Forms (Autodesk Fusion 360 design; units mm, degrees)
Autodesk Fusion 360 part; units mm, degrees
note: some values were not read from the file. Set by a fixed rule: which sketch regions a step uses.
sketch "Sketch1" plane through (0, 0, 0) normal (0, 0, 1) x (1, 0, 0)
  circle A0 centre (0, 0) radius 40
  circle A1 centre (150, 0) radius 40
  circle A2 centre (150, 0) radius 22.5
  line L0 (220, 40) -> (290, 40)
  line L1 (290, 40) -> (290, -30)
  line L2 (290, -30) -> (220, -30)
  line L3 (220, -30) -> (220, 40)
  line L4 (393.5132, 46.2887) -> (356.9124, 18.1157)
  line L5 (356.9124, 18.1157) -> (363.0105, -27.668)
  line L6 (363.0105, -27.668) -> (405.7094, -45.2787)
  line L7 (405.7094, -45.2787) -> (442.3102, -17.1057)
  line L8 (442.3102, -17.1057) -> (436.2121, 28.678)
  line L9 (436.2121, 28.678) -> (393.5132, 46.2887)
  point P0 (399.6113, 0.505)
  dimension "d1" = 80
  dimension "d2" = 80
  dimension "d3" = 45
  dimension "d4" = 70
  dimension "d5" = 70
  dimension "d6" = 40
  constraint coincident A0.centre origin
  constraint concentric A1 A2
  constraint horizontal L0
  constraint vertical L1
  constraint horizontal L2
  constraint vertical L3
  measures "d1" diameter of A0
  measures "d2" diameter of A1
  measures "d3" diameter of A2
  measures "d4" distance of L0.start L0.end
  measures "d5" distance of L0.start L2.end
  measures "d6" distance of P0 L9
extrude "Extrude1" add sketch "Sketch1" along normal blind 0.6 makes body 1 at (183.934, -3.105, 0) makes body 2 at (243.3333, 16.6667, 0) makes body 3 at (9.4847, -14.2223, 0) makes body 4 at (387.411, -8.886, 0)
sketch "Sketch2" plane through (0, 0, 0) normal (0, 0, 1) x (1, 0, 0)
  line L0 (-102.8513, 50) -> (-56.4512, -30.3672)
  line L1 (-56.4512, -30.3672) -> (-149.2513, -30.3672)
  line L2 (-149.2513, -30.3672) -> (-102.8513, 50)
  spline S0 degree 3 poles (-260.7978, 3.4174) (-243.8859, 0.3631) (-229.7421, -4.5389) (-219.4989, -12.0435) knots 0 0 0 0 1 1 1 1
  line L3 (-219.4989, -12.0435) -> (-224.2157, -12.0435)
  spline S1 degree 3 poles (-224.2157, -12.0435) (-234.8465, -6.8357) (-247.7436, -3.4645) (-262.3437, -1.4752) knots 0 0 0 0 1 1 1 1
  spline S2 degree 3 poles (-262.3437, -1.4752) (-262.9281, -1.3955) (-263.5204, -1.5157) (-264.038, -1.7987) knots 0 0 0 0 1 1 1 1
  spline S3 degree 3 poles (-264.038, -1.7987) (-267.9394, -3.9316) (-272.0672, -4.6023) (-276.5199, -4.8113) knots 0 0 0 0 1 1 1 1
  spline S4 degree 3 poles (-276.5199, -4.8113) (-279.9376, -4.9718) (-283.9097, -8.2703) (-284.0145, -9.2137) knots 0 0 0 0 1 1 1 1
  spline S5 degree 3 poles (-284.0145, -9.2137) (-286.3248, -30.0083) (-292.115, -40.2015) (-306.2361, -45.3236) knots 0 0 0 0 1 1 1 1
  spline S6 degree 3 poles (-306.2361, -45.3236) (-317.133, -48.2569) (-327.3208, -52.6393) (-337.0006, -58.0591) knots 0 0 0 0 1 1 1 1
  spline S7 degree 3 poles (-337.0006, -58.0591) (-336.8531, -67.2004) (-337.3497, -73.1816) (-338.2267, -77.2973) knots 0 0 0 0 1 1 1 1
  spline S8 degree 3 poles (-338.2267, -77.2973) (-338.2811, -77.5527) (-338.6377, -77.5743) (-338.7228, -77.3273) knots 0 0 0 0 1 1 1 1
  spline S9 degree 3 poles (-338.7228, -77.3273) (-340.0463, -73.4885) (-340.059, -67.9976) (-339.4115, -61.6754) knots 0 0 0 0 1 1 1 1
  spline S10 degree 3 poles (-339.4115, -61.6754) (-340.196, -70.3905) (-341.2782, -77.6979) (-342.7181, -83.3138) knots 0 0 0 0 1 1 1 1
  spline S11 degree 3 poles (-342.7181, -83.3138) (-342.7818, -83.562) (-343.1125, -83.6149) (-343.2471, -83.3969) knots 0 0 0 0 1 1 1 1
  spline S12 degree 3 poles (-343.2471, -83.3969) (-344.9354, -80.664) (-344.3802, -73.7091) (-341.8224, -62.9855) knots 0 0 0 0 1 1 1 1
  spline S13 degree 3 poles (-341.8224, -62.9855) (-343.6654, -68.0442) (-345.273, -72.8197) (-345.9627, -77.1363) knots 0 0 0 0 1 1 1 1
  spline S14 degree 3 poles (-345.9627, -77.1363) (-346.6868, -81.6681) (-347.3474, -85.3887) (-348.5401, -86.6625) knots 0 0 0 0 1 1 1 1
  spline S15 degree 3 poles (-348.5401, -86.6625) (-348.7985, -86.9386) (-349.2453, -86.9301) (-349.4925, -86.644) knots 0 0 0 0 1 1 1 1
  spline S16 degree 3 poles (-349.4925, -86.644) (-350.6585, -85.2949) (-350.8832, -82.2734) (-349.7887, -78.0269) knots 0 0 0 0 1 1 1 1
  spline S17 degree 3 poles (-349.7887, -78.0269) (-348.5261, -73.1287) (-346.4266, -68.1391) (-344.3905, -62.8804) knots 0 0 0 0 1 1 1 1
  spline S18 degree 3 poles (-344.3905, -62.8804) (-346.9247, -68.2647) (-349.2979, -72.9995) (-351.402, -76.6499) knots 0 0 0 0 1 1 1 1
  spline S19 degree 3 poles (-351.402, -76.6499) (-351.4977, -76.816) (-351.7419, -76.8027) (-351.8199, -76.6275) knots 0 0 0 0 1 1 1 1
  spline S20 degree 3 poles (-351.8199, -76.6275) (-352.271, -75.6135) (-352.5103, -74.3407) (-351.9899, -72.9432) knots 0 0 0 0 1 1 1 1
  spline S21 degree 3 poles (-351.9899, -72.9432) (-350.8238, -69.8118) (-348.3529, -65.5636) (-346.6966, -62.8804) knots 0 0 0 0 1 1 1 1
  spline S22 degree 3 poles (-346.6966, -62.8804) (-348.4004, -64.8165) (-350.018, -66.7369) (-351.5361, -68.6392) knots 0 0 0 0 1 1 1 1
  spline S23 degree 3 poles (-351.5361, -68.6392) (-351.6431, -68.7732) (-351.8603, -68.697) (-351.8581, -68.5254) knots 0 0 0 0 1 1 1 1
  spline S24 degree 3 poles (-351.8581, -68.5254) (-351.8238, -65.7106) (-348.2696, -62.1588) (-345.7532, -57.9018) knots 0 0 0 0 1 1 1 1
  spline S25 degree 3 poles (-345.7532, -57.9018) (-343.353, -53.8412) (-343.0694, -48.7587) (-343.0278, -43.5938) knots 0 0 0 0 1 1 1 1
  spline S26 degree 3 poles (-343.0278, -43.5938) (-342.8346, -36.7125) (-341.0335, -30.7038) (-337.6296, -25.5647) knots 0 0 0 0 1 1 1 1
  spline S27 degree 3 poles (-337.6296, -25.5647) (-339.0225, -27.1571) (-340.4289, -28.1941) (-341.8523, -28.5418) knots 0 0 0 0 1 1 1 1
  spline S28 degree 3 poles (-341.8523, -28.5418) (-342.2112, -28.6295) (-342.5542, -28.3294) (-342.4991, -27.9641) knots 0 0 0 0 1 1 1 1
  spline S29 degree 3 poles (-342.4991, -27.9641) (-341.9561, -24.3647) (-337.6367, -20.0679) (-333.2801, -15.7644) knots 0 0 0 0 1 1 1 1
  spline S30 degree 3 poles (-333.2801, -15.7644) (-338.7374, -21.2252) (-344.2145, -25.6888) (-349.7179, -28.8857) knots 0 0 0 0 1 1 1 1
  spline S31 degree 3 poles (-349.7179, -28.8857) (-349.9461, -29.0183) (-350.2082, -28.778) (-350.0965, -28.5389) knots 0 0 0 0 1 1 1 1
  spline S32 degree 3 poles (-350.0965, -28.5389) (-347.7567, -23.5322) (-342.0571, -19.1377) (-336.2153, -14.7685) knots 0 0 0 0 1 1 1 1
  spline S33 degree 3 poles (-336.2153, -14.7685) (-339.0427, -17.3429) (-342.3108, -19.242) (-345.5638, -21.431) knots 0 0 0 0 1 1 1 1
  spline S34 degree 3 poles (-345.5638, -21.431) (-349.1875, -23.8693) (-351.6975, -26.9643) (-356.2946, -27.6713) knots 0 0 0 0 1 1 1 1
  spline S35 degree 3 poles (-356.2946, -27.6713) (-356.6004, -27.7184) (-356.8157, -27.374) (-356.6379, -27.1208) knots 0 0 0 0 1 1 1 1
  spline S36 degree 3 poles (-356.6379, -27.1208) (-353.9362, -22.2172) (-346.509, -17.533) (-339.4126, -13.5629) knots 0 0 0 0 1 1 1 1
  spline S37 degree 3 poles (-339.4126, -13.5629) (-348.5941, -18.5484) (-357.9988, -24.0418) (-362.7798, -25.3474) knots 0 0 0 0 1 1 1 1
  spline S38 degree 3 poles (-362.7798, -25.3474) (-363.1677, -25.4533) (-363.538, -25.1083) (-363.4388, -24.7186) knots 0 0 0 0 1 1 1 1
  spline S39 degree 3 poles (-363.4388, -24.7186) (-362.6459, -21.6042) (-354.2725, -17.3356) (-344.3382, -12.8296) knots 0 0 0 0 1 1 1 1
  spline S40 degree 3 poles (-344.3382, -12.8296) (-353.2052, -16.5242) (-363.2289, -20.8213) (-366.6642, -21.6868) knots 0 0 0 0 1 1 1 1
  spline S41 degree 3 poles (-366.6642, -21.6868) (-368.0791, -22.1148) (-369.2325, -22.1652) (-370.2679, -22.045) knots 0 0 0 0 1 1 1 1
  spline S42 degree 3 poles (-370.2679, -22.045) (-370.7274, -21.9917) (-370.9442, -21.4371) (-370.6353, -21.0928) knots 0 0 0 0 1 1 1 1
  spline S43 degree 3 poles (-370.6353, -21.0928) (-367.6264, -17.7386) (-355.2227, -14.2376) (-345.9626, -10.7862) knots 0 0 0 0 1 1 1 1
  spline S44 degree 3 poles (-345.9626, -10.7862) (-355.4959, -13.5245) (-364.6122, -16.3755) (-370.4639, -17.8942) knots 0 0 0 0 1 1 1 1
  spline S45 degree 3 poles (-370.4639, -17.8942) (-371.8406, -18.1302) (-373.6743, -18.2066) (-375.3888, -17.9199) knots 0 0 0 0 1 1 1 1
  spline S46 degree 3 poles (-375.3888, -17.9199) (-375.812, -17.8491) (-375.9516, -17.3158) (-375.6267, -17.0354) knots 0 0 0 0 1 1 1 1
  spline S47 degree 3 poles (-375.6267, -17.0354) (-372.1238, -14.0115) (-360.9311, -11.379) (-348.793, -8.7947) knots 0 0 0 0 1 1 1 1
  spline S48 degree 3 poles (-348.793, -8.7947) (-363.3832, -11.6385) (-377.3886, -14.4346) (-386.0111, -16.7904) knots 0 0 0 0 1 1 1 1
  spline S49 degree 3 poles (-386.0111, -16.7904) (-386.3201, -16.8749) (-386.634, -16.9416) (-386.952, -16.9802) knots 0 0 0 0 1 1 1 1
  spline S50 degree 3 poles (-386.952, -16.9802) (-389.2926, -17.2641) (-391.9533, -17.3016) (-394.7602, -17.2264) knots 0 0 0 0 1 1 1 1
  spline S51 degree 3 poles (-394.7602, -17.2264) (-395.209, -17.2144) (-395.3665, -16.6235) (-394.9808, -16.3938) knots 0 0 0 0 1 1 1 1
  spline S52 degree 3 poles (-394.9808, -16.3938) (-393.6599, -15.6072) (-391.2932, -14.4235) (-388.1521, -13.7737) knots 0 0 0 0 1 1 1 1
  spline S53 degree 3 poles (-388.1521, -13.7737) (-374.4736, -10.9436) (-354.6944, -6.3006) (-354.5578, -6.0695) knots 0 0 0 0 1 1 1 1
  spline S54 degree 3 poles (-354.5578, -6.0695) (-354.3742, -5.7602) (-393.7305, -13.0345) (-402.8093, -15.0947) knots 0 0 0 0 1 1 1 1
  spline S55 degree 3 poles (-402.8093, -15.0947) (-404.4616, -15.4697) (-406.1476, -15.6754) (-407.8417, -15.7015) knots 0 0 0 0 1 1 1 1
  spline S56 degree 3 poles (-407.8417, -15.7015) (-409.7184, -15.7304) (-411.4213, -15.6873) (-412.6827, -15.461) knots 0 0 0 0 1 1 1 1
  spline S57 degree 3 poles (-412.6827, -15.461) (-413.1591, -15.3756) (-413.2304, -14.7209) (-412.7835, -14.535) knots 0 0 0 0 1 1 1 1
  spline S58 degree 3 poles (-412.7835, -14.535) (-403.8503, -10.8205) (-379.2892, -6.9049) (-357.8597, -3.03) knots 0 0 0 0 1 1 1 1
  spline S59 degree 3 poles (-357.8597, -3.03) (-379.6178, -5.5238) (-400.1391, -8.7621) (-418.2351, -13.459) knots 0 0 0 0 1 1 1 1
  spline S60 degree 3 poles (-418.2351, -13.459) (-421.5535, -14.0118) (-424.5181, -13.9609) (-427.037, -13.1496) knots 0 0 0 0 1 1 1 1
  spline S61 degree 3 poles (-427.037, -13.1496) (-427.4679, -13.0108) (-427.5166, -12.4193) (-427.1184, -12.2038) knots 0 0 0 0 1 1 1 1
  spline S62 degree 3 poles (-427.1184, -12.2038) (-419.0775, -7.8516) (-387.5805, -4.0579) (-363.2051, -0.0943) knots 0 0 0 0 1 1 1 1
  spline S63 degree 3 poles (-363.2051, -0.0943) (-386.7089, -2.1136) (-374.4342, 1.1504) (-429.241, -10.2616) knots 0 0 0 0 1 1 1 1
  spline S64 degree 3 poles (-429.241, -10.2616) (-431.8767, -10.8397) (-434.9447, -10.818) (-438.1939, -10.5444) knots 0 0 0 0 1 1 1 1
  spline S65 degree 3 poles (-438.1939, -10.5444) (-438.8722, -10.4873) (-439.0643, -9.5883) (-438.4683, -9.2593) knots 0 0 0 0 1 1 1 1
  spline S66 degree 3 poles (-438.4683, -9.2593) (-429.0555, -4.0638) (-393.5502, -0.7209) (-367.0308, 3.2601) knots 0 0 0 0 1 1 1 1
  spline S67 degree 3 poles (-367.0308, 3.2601) (-374.8305, 5.3234) (-410.4613, -2.0434) (-440.4561, -7.4314) knots 0 0 0 0 1 1 1 1
  spline S68 degree 3 poles (-440.4561, -7.4314) (-443.1112, -7.9083) (-445.5556, -7.584) (-447.6828, -6.9507) knots 0 0 0 0 1 1 1 1
  spline S69 degree 3 poles (-447.6828, -6.9507) (-448.207, -6.7947) (-448.2438, -6.0617) (-447.7389, -5.8517) knots 0 0 0 0 1 1 1 1
  spline S70 degree 3 poles (-447.7389, -5.8517) (-430.384, 1.3653) (-404.062, 4.6451) (-376.0451, 6.6141) knots 0 0 0 0 1 1 1 1
  spline S71 degree 3 poles (-376.0451, 6.6141) (-376.9414, 7.4241) (-377.4204, 8.2626) (-375.9402, 9.2346) knots 0 0 0 0 1 1 1 1
  spline S72 degree 3 poles (-375.9402, 9.2346) (-371.4152, 10.048) (-364.1924, 10.3178) (-356.4967, 10.4925) knots 0 0 0 0 1 1 1 1
  spline S73 degree 3 poles (-356.4967, 10.4925) (-367.1624, 10.6072) (-376.8832, 11.2482) (-384.3663, 13.1344) knots 0 0 0 0 1 1 1 1
  spline S74 degree 3 poles (-384.3663, 13.1344) (-384.8788, 13.2636) (-384.9042, 13.9783) (-384.4046, 14.1505) knots 0 0 0 0 1 1 1 1
  spline S75 degree 3 poles (-384.4046, 14.1505) (-379.9195, 15.6966) (-370.8806, 16.1514) (-358.855, 15.8906) knots 0 0 0 0 1 1 1 1
  spline S76 degree 3 poles (-358.855, 15.8906) (-373.5318, 16.4635) (-385.9218, 17.6108) (-392.235, 20.2839) knots 0 0 0 0 1 1 1 1
  spline S77 degree 3 poles (-392.235, 20.2839) (-392.7657, 20.5085) (-392.6939, 21.2829) (-392.1298, 21.4002) knots 0 0 0 0 1 1 1 1
  spline S78 degree 3 poles (-392.1298, 21.4002) (-384.1009, 23.069) (-374.3025, 22.7026) (-363.7298, 21.4461) knots 0 0 0 0 1 1 1 1
  spline S79 degree 3 poles (-363.7298, 21.4461) (-377.4672, 22.9823) (-389.4616, 25.0524) (-397.8117, 28.2399) knots 0 0 0 0 1 1 1 1
  spline S80 degree 3 poles (-397.8117, 28.2399) (-398.3914, 28.4611) (-398.2929, 29.3109) (-397.6782, 29.3959) knots 0 0 0 0 1 1 1 1
  spline S81 degree 3 poles (-397.6782, 29.3959) (-390.0149, 30.4568) (-380.5332, 29.5894) (-370.0712, 27.6827) knots 0 0 0 0 1 1 1 1
  spline S82 degree 3 poles (-370.0712, 27.6827) (-383.4488, 29.6324) (-394.7957, 32.9589) (-403.128, 38.3296) knots 0 0 0 0 1 1 1 1
  spline S83 degree 3 poles (-403.128, 38.3296) (-403.4817, 38.5576) (-403.3163, 39.1078) (-402.8956, 39.0977) knots 0 0 0 0 1 1 1 1
  spline S84 degree 3 poles (-402.8956, 39.0977) (-395.0473, 38.9082) (-384.3504, 36.5793) (-371.7479, 32.8192) knots 0 0 0 0 1 1 1 1
  spline S85 degree 3 poles (-371.7479, 32.8192) (-387.9509, 38.3146) (-399.2799, 43.2259) (-404.9262, 47.4558) knots 0 0 0 0 1 1 1 1
  spline S86 degree 3 poles (-404.9262, 47.4558) (-405.5172, 47.8987) (-405.2174, 48.8457) (-404.4791, 48.8639) knots 0 0 0 0 1 1 1 1
  spline S87 degree 3 poles (-404.4791, 48.8639) (-392.1436, 49.1686) (-369.0639, 37.0794) (-347.063, 27.6827) knots 0 0 0 0 1 1 1 1
  spline S88 degree 3 poles (-347.063, 27.6827) (-336.4661, 23.1566) (-327.4168, 18.0243) (-320.3337, 11.5931) knots 0 0 0 0 1 1 1 1
  spline S89 degree 3 poles (-320.3337, 11.5931) (-317.2166, 8.7627) (-316.6539, 3.5021) (-313.9922, 1.583) knots 0 0 0 0 1 1 1 1
  spline S90 degree 3 poles (-313.9922, 1.583) (-312.4731, 0.4877) (-309.3016, 0.561) (-308.6989, 1.4257) knots 0 0 0 0 1 1 1 1
  spline S91 degree 3 poles (-308.6989, 1.4257) (-300.6658, 12.9513) (-294.6695, 20.6621) (-284.7477, 20.7647) knots 0 0 0 0 1 1 1 1
  spline S92 degree 3 poles (-284.7477, 20.7647) (-276.2498, 20.8525) (-268.2813, 15.7079) (-260.7965, 3.417) knots 0 0 0 0 1 1 1 1
  line L4 (-260.7965, 3.417) -> (-260.7978, 3.4174)
extrude "Extrude2" add sketch "Sketch2" along normal blind 0.6 separate body contours L0 L1 L2 | S0 L3 S1 S2 S3 S4 S5 S6 S7 S8 S9 S10 S11 S12 S13 S14 S15 S16 S17 S18 S19 S20 S21 S22 S23 S24 S25 S26 S27 S28 S29 S30 S31 S32 S33 S34 S35 S36 S37 S38 S39 S40 S41 S42 S43 S44 S45 S46 S47 S48 S49 S50 S51 S52 S53 S54 S55 S56 S57 S58 S59 S60 S61 S62 S63 S64 S65 S66 S67 S68 S69 S70 S71 S72 S73 S74 S75 S76 S77 S78 S79 S80 S81 S82 S83 S84 S85 S86 S87 S88 S89 S90 S91 S92 makes body 5 at (-102.8512, -3.5781, 0) makes body 6 at (-313.6214, -18.4264, 0)
